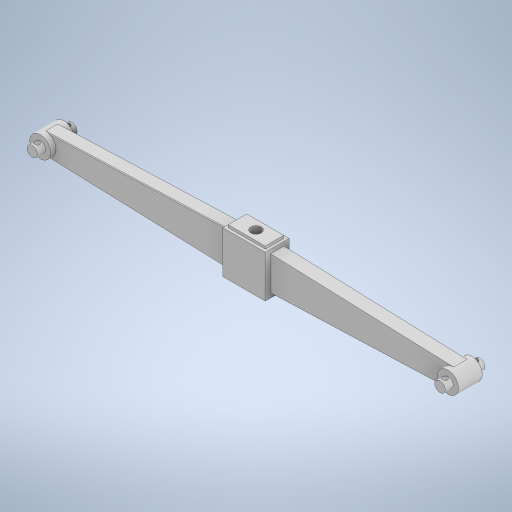
# Autodesk Inventor part: HUDSON-1-11-AXLE BROX SPRING
Saved by Autodesk Inventor 2024.2 (Build 282272000, 272)
## iProperties
Created: 2024-10-08
Part Number: HUDSON-1-11-AXLE BROX SPRING
Material: Generic
Document SubType Name: Modeling
Designer: Jimena Brenes
Density: 1 g/cm^3
Appearance: Default
Author: Jimena Brenes
Autodesk Inventor part; units mm, degrees
ref_plane "YZ Plane" through (0, 0, 0) normal (1, 0, 0) x (0, 1, 0)
ref_plane "XY Plane" through (0, 0, 0) normal (0, 0, 1) x (1, 0, 0)
sketch "Sketch1" plane through (0, 0, 0) normal (0, 0, 1) x (1, 0, 0)
  circle A0 centre (0, 0) radius 4
  circle A1 centre (0, 0) radius 2
  line L0 (69, 8) -> (85, 8)
  line L1 (85, 8) -> (85, -8)
  line L2 (85, -8) -> (69, -8)
  line L3 (69, -8) -> (69, 8)
  line L4 (0, 0) -> (147, 0) construction
  line L5 (-0.145, -3.9974) -> (69, -6.5062)
  line L6 (-0.1446, 3.9974) -> (69, 6.499)
  line L7 (70, 8) -> (70, 9)
  line L8 (70, 9) -> (84, 9)
  line L9 (84, 9) -> (84, 8)
  line L10 (77, 38) -> (77, -54) construction
  circle A2 centre (154, 0) radius 4
  circle A3 centre (154, 0) radius 2
  line L11 (154.145, -3.9974) -> (85, -6.5062)
  line L12 (154.1446, 3.9974) -> (85, 6.499)
  point P0 (70, 8.5)
  point P1 (84, 8.5)
  dimension "d2" = 8
  dimension "d3" = 4
  dimension "d4" = 16
  dimension "d5" = 16
  dimension "d6" = 8
  dimension "d7" = 69
  dimension "d8" = 4.15
  dimension "d9" = 1.5
  dimension "d10" = 17
  dimension "d11" = 14
  dimension "d12" = 1
  dimension "d13" = 8
  constraints: 26 end point, 6 symmetric about line, 4 centre point, 4 point on circle, 4 point on line, 3 coincident, 3 parallel, 2 horizontal, 2 midpoint, 2 perpendicular, 2 tangent, 2 vertical, 2 other
  measures "d2" diameter of A0
  measures "d3" diameter of A1
  measures "d4" distance between parallel lines of L2 L0
  measures "d5" distance between parallel lines of L1 L3
  measures "d6" distance between parallel lines of L4 L2
  measures "d7" distance from line of point (0, 0) L3
  measures "d8" angle of L5 L6
  measures "d9" distance from line of L0.start L6
  measures "d10" distance between parallel lines of L2 L8
  measures "d11" distance of point (70, 8.5) point (84, 8.5)
  measures "d12" horizontal distance of L0.start point (70, 8.5)
  measures "d13" distance between parallel lines of L3 L10
extrude "Extrusion1" add sketch "Sketch1" along normal mid plane 9 contours L3 L0 L1 L2
extrude "Extrusion2" add sketch "Sketch1" along normal mid plane 7 contours L7 L8 L9 L0
extrude "Extrusion3" add sketch "Sketch1" along normal mid plane 5 contours A0 L6 L3 L5 | L1 L12 A2 L11
extrude "Extrusion4" add sketch "Sketch1" along normal mid plane 15 contours A1 | A3
extrude "Extrusion5" add sketch "Sketch1" along normal mid plane 9 contours A0 | A2 | A1 | A3
chamfer "Chamfer1" distance 0.25 angle 45 6 edges at (34.4277, 5.2482, 2.5) (34.4277, 5.2482, -2.5) (34.4275, -5.2518, 2.5) (119.5725, -5.2518, -2.5) (34.4275, -5.2518, -2.5) (119.5725, -5.2518, 2.5)
ref_plane "Work Plane1" through (0, 5, 0) normal (0, 1, 0) x (-1, 0, 0)
sketch "Sketch2" plane through (0, 5, 0) normal (0, 1, 0) x (-1, 0, 0)
  circle A0 centre (0, -5.75) radius 1
  circle A1 centre (0, 5.75) radius 1
  line L0 (2, 7.5) -> (-2, 7.5) projected
  line L1 (-2, -7.5) -> (2, -7.5) projected
  line L2 (-77, -9) -> (-77, 47) construction
  line L3 (-85, -4.5) -> (-85, 4.5) projected
  circle A2 centre (-154, -5.75) radius 1
  circle A3 centre (-154, 5.75) radius 1
  point P0 (0, 0)
  point P1 (-154, 0)
  point P2 (-152, 7.5)
  point P3 (-152, -7.5)
  dimension "d28" = 2
  dimension "d29" = 2
  dimension "d30" = 11.5
  dimension "d32" = 1.75
  dimension "d33" = 1.75
  dimension "d34" = 8
  dimension "d35" = 2
  constraints: 5 symmetric about line, 4 centre point, 2 end point, 1 vertical, 2 other
  measures "d28" diameter of A0
  measures "d29" diameter of A1
  measures "d30" distance of A1.centre A0.centre
  measures "d32" distance from line of L0 A1.centre
  measures "d33" distance from line of L1 A0.centre
  measures "d34" distance between parallel lines of L3 L2
  measures "d35" diameter of A3
hole "Hole1" at (0, 5, -5.75) at (0, 5, 5.75) at (154, 5, 5.75) at (154, 5, -5.75) direction (0, -1, 0) diameter 2 end through all
sketch "Sketch3" plane through (70, 9, 3.5) normal (0, 1, 0) x (1, 0, 0)
  circle A0 centre (7, 3.5) radius 2
  line L0 (15, 8) -> (15, -1) projected
  line L1 (-1, 8) -> (15, 8) projected
  point P0 (-70, 3.5)
  dimension "d43" = 4
  dimension "d44" = 8
  dimension "d45" = 4.5
  constraints: 1 centre point
  measures "d43" diameter of A0
  measures "d44" distance from line of L0 A0.centre
  measures "d45" distance from line of L1 A0.centre
hole "Hole2" at (77, 9, 0) direction (0, -1, 0) diameter 4 end through all
body "Solid1"
